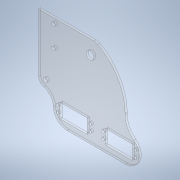
# Autodesk Inventor part: Intake Sides V5_servo
Saved by Autodesk Inventor 2022 (Build 260153000, 153)
## iProperties
Created: 2022-10-16
Part Number: Intake Sides V5_servo
Material: Polycarbonate, Clear
Document SubType Name: Modeling
Designer: matt
Density: 1.2 g/cm^3
Appearance: Polycarbonate - Clear
Mass: 60.255 g
Surface Area: 348.282 cm^2
Volume: 50.2125 cm^3
Author: matt
Autodesk Inventor part; units mm, degrees
ref_plane "YZ Plane" through (0, 0, 0) normal (1, 0, 0) x (0, 1, 0)
ref_plane "XZ Plane" through (0, 0, 0) normal (0, 1, 0) x (-1, 0, 0)
ref_plane "XY Plane" through (0, 0, 0) normal (0, 0, 1) x (1, 0, 0)
sketch "Sketch1" plane through (0, 0, 0) normal (0, 0, 1) x (1, 0, 0)
  line L0 (131.6573, -73.5015) -> (131.6573, -71.6343)
  arc A0 (131.6573, -71.6343) -> (90.0875, -1.2951) centre (51.3628, -71.6343) ccw
  arc A1 (90.0875, -1.2951) -> (83.8803, 0.1854) centre (84.3001, -11.8073) ccw
  line L1 (83.8803, 0.1854) -> (0.0078, 0.1927)
  line L2 (0.0078, 0.1927) -> (0, -88.6441)
  arc A2 (0, -88.6441) -> (8.2038, -98.4815) centre (10, -88.6441) ccw
  circle A3 centre (121.1882, -82.4439) radius 3.3
  arc A4 (146.0697, -114.2869) -> (148.3706, -110.4201) centre (147.2459, -112.3689) ccw
  circle A5 centre (97.7459, -122.3689) radius 2.25
  circle A6 centre (97.7459, -112.3689) radius 2.25
  circle A7 centre (78.1758, -122.3689) radius 2.25
  arc A8 (146.0697, -124.2869) -> (148.3706, -120.4201) centre (147.2459, -122.3689) ccw
  circle A9 centre (22.6171, -8.5119) radius 2.8
  circle A10 centre (22.6171, -40.5119) radius 2.8
  circle A11 centre (28.6758, -122.3689) radius 2.25
  circle A12 centre (28.6758, -112.3689) radius 2.25
  circle A13 centre (78.1758, -112.3689) radius 2.25
  circle A14 centre (10, -88.6441) radius 3.3
  line L3 (73.0605, -128.2915) -> (33.527, -128.2915)
  arc A15 (32.527, -127.2915) -> (33.527, -128.2915) centre (33.527, -127.2915) ccw
  line L4 (32.527, -127.2915) -> (32.527, -107.4915)
  arc A16 (33.527, -106.4915) -> (32.527, -107.4915) centre (33.527, -107.4915) ccw
  line L5 (33.527, -106.4915) -> (73.0605, -106.4915)
  arc A17 (74.0605, -107.4915) -> (73.0605, -106.4915) centre (73.0605, -107.4915) ccw
  line L6 (74.0605, -107.4915) -> (74.0605, -127.2915)
  arc A18 (73.0605, -128.2915) -> (74.0605, -127.2915) centre (73.0605, -127.2915) ccw
  line L7 (142.1306, -128.2915) -> (102.597, -128.2915)
  arc A19 (101.597, -127.2915) -> (102.597, -128.2915) centre (102.597, -127.2915) ccw
  line L8 (101.597, -127.2915) -> (101.597, -107.4915)
  arc A20 (102.597, -106.4915) -> (101.597, -107.4915) centre (102.597, -107.4915) ccw
  line L9 (102.597, -106.4915) -> (142.1306, -106.4915)
  arc A21 (143.1306, -107.4915) -> (142.1306, -106.4915) centre (142.1306, -107.4915) ccw
  line L10 (143.1306, -107.4915) -> (143.1306, -127.2915)
  arc A22 (142.1306, -128.2915) -> (143.1306, -127.2915) centre (142.1306, -127.2915) ccw
  circle A23 centre (147.2459, -112.3689) radius 2.25
  circle A24 centre (147.2459, -122.3689) radius 2.25
  line L11 (28.6758, -112.3689) -> (147.2459, -112.3689) construction
  line L12 (28.6758, -122.3689) -> (147.2459, -122.3689) construction
  circle A25 centre (43.3788, -117.3688) radius 6
  circle A26 centre (22.6171, -40.5119) radius 2.8 projected
  circle A27 centre (22.6171, -8.5119) radius 2.8 projected
  circle A28 centre (132.2788, -117.3688) radius 6
  circle A29 centre (78.1758, -21.998) radius 3.25
  circle A30 centre (78.1758, -21.998) radius 6
  arc A31 (132.2788, -138.3688) -> (145.0698, -100.7137) centre (132.2788, -117.3688) ccw
  arc A32 (22.3815, -117.7081) -> (8.2038, -98.4815) centre (1.805, -118.0406) ccw
  line L13 (43.3788, -138.3688) -> (132.2788, -138.3688)
  arc A33 (131.6573, -73.5015) -> (145.0698, -100.7137) centre (165.9686, -73.5015) ccw
  arc A34 (22.3815, -117.7081) -> (43.3788, -138.3688) centre (43.3788, -117.3688) ccw
  point P0 (0, 0)
  point P1 (58.8546, -117.3689)
  dimension "d2" = 49.5
  dimension "d3" = 49.5
  dimension "d4" = 49.5
  dimension "d5" = 49.5
  dimension "d6" = 10
  dimension "d7" = 12
  dimension "d10" = 88.9
  dimension "d11" = 42
  dimension "d13" = 10.8518
  dimension "d14" = 10.8518
  dimension "d15" = 4.1153
  dimension "d16" = 4.1153
  dimension "d17" = 4.1153
  dimension "d18" = 78.17
  constraints: 34 point on circle, 33 centre point, 28 end point, 5 coincident, 4 point on line, 3 tangent, 2 concentric, 2 perpendicular, 1 horizontal
  measures "d2" distance of A13.centre L11.start
  measures "d3" distance of A7.centre L12.start
  measures "d4" distance of L12.end A5.centre
  measures "d5" distance of L11.end A6.centre
  measures "d6" distance of L12.start L11.start
  measures "d7" diameter of A30
  measures "d10" distance of A28.centre A25.centre
  measures "d11" diameter of A31
  measures "d13" distance from line of L4 A25.centre
  measures "d14" distance from line of L10 A28.centre
  measures "d15" distance from line of L6 A13.centre
  measures "d16" distance from line of L10 L11.end
  measures "d17" distance from line of L10 L12.end
  measures "d18" distance from line of L2 A30.centre
extrude "Extrusion1" add sketch "Sketch1" along normal blind 3.175 contours A33 A31 L13 A34 A32 A2 L2 L1 A1 A0 L0 | A14
equation "\"d14\" = d13"
equation "\"d16\" = d15"
equation "\"d17\" = d15"
body "Solid1"
